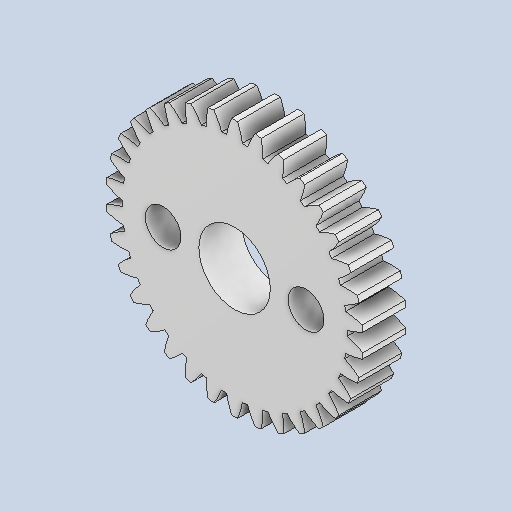
# Autodesk Inventor part: 平歯車1
Saved by Autodesk Inventor 2025.2 (Build 292293000, 293)
## iProperties
CustomPartVersion: 1
Created: 2025-01-10
Part Number: 平歯車1
Material: ABS プラスチック
Document SubType Name: Modeling
Designer: haruy
Categories: <?xml version="1.0" encoding="UTF-16"?> <MemberInstance><Categories><FamilyTemplate><FamilyTemplateParameter ValueType="xs:double" Id="1" ObjectReferenceKey="da_z" ObjectType="kUserParameterObject"/><FamilyTemplateParameter ValueType="xs:double" Id="2" ObjectReferenceKey="da_b" ObjectType="kUserParameterObject"/><FamilyTemplateParameter ValueType="xs:double" Id="3" ObjectReferenceKey="da_beta" ObjectType="kUserParameterObject"/><FamilyTemplateParameter ValueType="xs:double" Id="4" ObjectReferenceKey="da_da" ObjectType="kUserParameterObject"/><FamilyTemplateParameter ValueType="xs:double" Id="5" ObjectReferenceKey="da_aw" ObjectType="kUserParameterObject"/><FamilyTemplateParameter ValueType="xs:string" Id="6" ObjectReferenceKey="EAIAABAAAACIAQAAAAAAAIAAAAAAAAAA" ObjectType="83910656" SubObjectId="SurfaceGeometry"/></FamilyTemplate><ParamToTemplateMap><ParamToTemplate CategoryParameter="//CategoryParameter[@InternalName='046C89C9-8512-4d59-83FE-43B91F4F132A']" TemplateParameter="1"/><ParamToTemplate CategoryParameter="//CategoryParameter[@InternalName='2552DF32-E462-4b46-AEBF-C6C7768E72AC']" TemplateParameter="2"/><ParamToTemplate CategoryParameter="//CategoryParameter[@InternalName='C9EE641D-15FC-4fae-A226-E94C4372FDD7']" TemplateParameter="3"/><ParamToTemplate><ParamToTemplate CategoryParameter="//CategoryParameter[@InternalName='00B6519A-459B-49c7-AD84-2E56D39A5744']" ConstantValue="0.000000"/></ParamToTemplate><ParamToTemplate><ParamToTemplate CategoryParameter="//CategoryParameter[@InternalName='04B31F0E-C7A6-4894-AA32-9629BEFACF47']" ConstantValue="1.000000"/></ParamToTemplate><ParamToTemplate><ParamToTemplate CategoryParameter="//CategoryParameter[@InternalName='43CBEC2E-7847-49e7-A936-2F7889FCB2D9']" ConstantValue="0.250000"/></ParamToTemplate><ParamToTemplate><ParamToTemplate CategoryParameter="//CategoryParameter[@InternalName='B1EFC894-105D-4ebd-86BF-FA20ED196853']" ConstantValue="0.350000"/></ParamToTemplate><ParamToTemplate><ParamToTemplate CategoryParameter="//CategoryParameter[@InternalName='51175063-3D10-4879-93E8-6246FE8B403D']" ConstantValue="2060000000.000000"/></ParamToTemplate><ParamToTemplate><ParamToTemplate CategoryParameter="//CategoryParameter[@InternalName='A3A52E27-4454-46a9-B0BD-C932399B70AF']" ConstantValue="0.300000"/></ParamToTemplate><ParamToTemplate><ParamToTemplate CategoryParameter="//CategoryParameter[@InternalName='91B76062-C214-41d9-B1B9-14D2AB99603D']" ConstantValue="0.100000"/></ParamToTemplate><ParamToTemplate><ParamToTemplate CategoryParameter="//CategoryParameter[@InternalName='374E806E-8B8A-4dda-A9AA-1039D6500AD2']" ConstantValue="10.000000"/></ParamToTemplate><ParamToTemplate><ParamToTemplate CategoryParameter="//CategoryParameter[@InternalName='2D373A89-B862-43d6-8D0B-0CBF12AB9F6C']" ConstantValue="0.349066"/></ParamToTemplate><ParamToTemplate CategoryParameter="//CategoryParameter[@InternalName='37777632-D6A2-4fac-9D53-DB8ACD95C989']" TemplateParameter="4"/><ParamToTemplate CategoryParameter="//CategoryParameter[@InternalName='FD1017F1-B727-4f7e-9707-0F86F1FF9423']" TemplateParameter="5"/><ParamToTemplate><ParamToTemplate CategoryParameter="//CategoryParameter[@InternalName='9E1B4470-B2D3-4ff1-B813-535BB4CDF51A']" ConstantValue="3520000.000000"/></ParamToTemplate><ParamToTemplate><ParamToTemplate CategoryParameter="//CategoryParameter[@InternalName='F8452263-BFF6-458c-9FB1-07C4B99E95CD']" ConstantValue="11400000.000000"/></ParamToTemplate><ParamToTemplate><ParamToTemplate CategoryParameter="//CategoryParameter[@InternalName='3E3BB259-FD49-497f-8171-6EBC954A3479']" ConstantValue="2.000000"/></ParamToTemplate><ParamToTemplate CategoryParameter="//CategoryParameter[@InternalName='27C3BAF2-7550-4e4b-AE2C-0DB134B7D9B7']" TemplateParameter="6"/></ParamToTemplateMap><Category DisplayName="Gear" InternalName="DC85795E-93AB-48d5-8EEE-5A27447B64BD" Mnemonic="Gear"><CategoryParameter DisplayName="z" InternalName="046C89C9-8512-4d59-83FE-43B91F4F132A" Mnemonic="z"/><CategoryParameter DisplayName="b" InternalName="2552DF32-E462-4b46-AEBF-C6C7768E72AC" Mnemonic="b"/><CategoryParameter DisplayName="||b|" InternalName="C9EE641D-15FC-4fae-A226-E94C4372FDD7" Mnemonic="beta"/><CategoryParameter DisplayName="x" InternalName="00B6519A-459B-49c7-AD84-2E56D39A5744" Mnemonic="x"/><CategoryParameter DisplayName="a*" InternalName="04B31F0E-C7A6-4894-AA32-9629BEFACF47" Mnemonic="a"/><CategoryParameter DisplayName="c*" InternalName="43CBEC2E-7847-49e7-A936-2F7889FCB2D9" Mnemonic="c"/><CategoryParameter DisplayName="r|.f|*" InternalName="B1EFC894-105D-4ebd-86BF-FA20ED196853" Mnemonic="rf"/><CategoryParameter DisplayName="E" InternalName="51175063-3D10-4879-93E8-6246FE8B403D" Mnemonic="E"/><CategoryParameter DisplayName="||m|" InternalName="A3A52E27-4454-46a9-B0BD-C932399B70AF" Mnemonic="mi"/><Category DisplayName="SpurGear" InternalName="26C5A22E-A91E-4dfd-A3B3-23CCAFAE1764" Mnemonic="SpurGear"><CategoryParameter DisplayName="m" InternalName="91B76062-C214-41d9-B1B9-14D2AB99603D" Mnemonic="m"/><CategoryParameter DisplayName="P" InternalName="374E806E-8B8A-4dda-A9AA-1039D6500AD2" Mnemonic="PP"/><CategoryParameter DisplayName="||a|" InternalName="2D373A89-B862-43d6-8D0B-0CBF12AB9F6C" Mnemonic="alpha"/><CategoryParameter DisplayName="d|.a|" InternalName="37777632-D6A2-4fac-9D53-DB8ACD95C989" Mnemonic="da"/><CategoryParameter DisplayName="a|.w|" InternalName="FD1017F1-B727-4f7e-9707-0F86F1FF9423" Mnemonic="aw"/><CategoryParameter DisplayName="||s||.Flim|" InternalName="9E1B4470-B2D3-4ff1-B813-535BB4CDF51A" Mnemonic="sFlim"/><CategoryParameter DisplayName="||s||.Hlim|" InternalName="F8452263-BFF6-458c-9FB1-07C4B99E95CD" Mnemonic="sHlim"/><CategoryParameter DisplayName="タイプ" InternalName="3E3BB259-FD49-497f-8171-6EBC954A3479" Mnemonic="type"/><CategoryParameter DisplayName="PitchDiameter" InternalName="27C3BAF2-7550-4e4b-AE2C-0DB134B7D9B7" Mnemonic="IDS_PITCHDIAM"/></Category></Category></Categories></MemberInstance>
Density: 1.06 g/cm^3
Appearance: 滑らか - 白
Author: haruy
Autodesk Inventor part; units mm, degrees
sketch "Sketch1" plane through (0, 0, 0) normal (0, 0, 1) x (1, 0, 0)
  circle A0 centre (0, 0) radius 18
  dimension "d0" = 36
  constraints: 1 centre point
  measures "d0" diameter of A0
extrude "Extrusion1" add sketch "Sketch1" along normal blind 6
ref_plane "Work Plane2" through (0, 0, 3) normal (0, 0, 1) x (1, 0, 0)
sketch "Sketch2" plane through (0, 0, 0) normal (0, 0, -1) x (-1, 0, 0)
  circle A0 centre (0, 0) radius 18 projected
  circle A1 centre (0, 0) radius 17
  dimension "d3" = 34
  constraints: 1 centre point, 1 coincident
  measures "d3" diameter of A1
surface extrude "ピッチ円直径" sketch "Sketch2" against normal through all shown no curves A1
ref_plane "Work Plane8" through (0, 0, 0) normal (0.9957342, 0.0922684, 0) x (0, 0, 1)
ref_plane "Work Plane9" through (0, 0, 0) normal (1, 0, 0) x (0, 1, 0)
spur gear teeth "平歯車" teeth 34 pitch diameter 34 tip diameter 36 root diameter 31.5 face width 6 start plane through (0, 0, 0) normal (0, 0, -1) x (-1, 0, 0)
sketch "スケッチ3" plane through (0, 0, 6) normal (0, 0, 1) x (1, 0, 0)
  circle A0 centre (0, 0) radius 5
  circle A1 centre (0, 0) radius 10
  circle A2 centre (-10, 0) radius 2.5
  circle A3 centre (10, 0) radius 2.5
  dimension "d50" = 20
  dimension "d49" = 10
  dimension "d51" = 5
  dimension "d54" = 360
  constraints: 3 centre point, 2 coincident, 1 horizontal alignment, 7 other
  measures "d49" diameter of A0
  measures "d51" diameter of A2
extrude "押し出し2" cut sketch "スケッチ3" against normal blind 10 contours A0 | A1 A3 | A1 A3 | A2 A1 | A1 A2
sketch "スケッチ4" plane through (0, 0, 6) normal (0, 0, 1) x (1, 0, 0)
  circle A0 centre (10, 0) radius 2.5 projected
  circle A1 centre (-10, 0) radius 2.5 projected
  circle A2 centre (0, 0) radius 5 projected
  arc A3 (-3.7153, 17.6124) -> (-3.9591, 15.2443) centre (6.5578, 15.358) ccw projected
  arc A4 (-3.9591, 15.2443) -> (-4.6589, 15.0452) centre (0, 0) ccw projected
  arc A5 (-4.6589, 15.0452) -> (-6.1129, 16.9302) centre (-13.6605, 9.6054) ccw projected
  arc A6 (-6.1129, 16.9302) -> (-6.8883, 16.6298) centre (0, 0) ccw projected
  arc A7 (-6.8883, 16.6298) -> (-6.6929, 14.2572) centre (3.6241, 16.3015) ccw projected
  arc A8 (-6.6929, 14.2572) -> (-7.3442, 13.9329) centre (0, 0) ccw projected
  arc A9 (-7.3442, 13.9329) -> (-9.1198, 15.5187) centre (-15.1929, 6.9317) ccw projected
  arc A10 (-9.1198, 15.5187) -> (-9.8267, 15.081) centre (0, 0) ccw projected
  arc A11 (-9.8267, 15.081) -> (-9.1987, 12.7847) centre (0.567, 16.6898) ccw projected
  arc A12 (-9.1987, 12.7847) -> (-9.7793, 12.3462) centre (0, 0) ccw projected
  arc A13 (-9.7793, 12.3462) -> (-11.816, 13.5787) centre (-16.2079, 4.022) ccw projected
  arc A14 (-11.816, 13.5787) -> (-12.4305, 13.0185) centre (0, 0) ccw projected
  arc A15 (-12.4305, 13.0185) -> (-11.3912, 10.8767) centre (-2.5094, 16.5098) ccw projected
  arc A16 (-11.3912, 10.8767) -> (-11.8814, 10.339) centre (0, 0) ccw projected
  arc A17 (-11.8814, 10.339) -> (-14.1099, 11.1763) centre (-16.6709, 0.9753) ccw projected
  arc A18 (-14.1099, 11.1763) -> (-14.611, 10.5127) centre (0, 0) ccw projected
  arc A19 (-14.611, 10.5127) -> (-13.1958, 8.5984) centre (-5.5003, 15.7676) ccw projected
  arc A20 (-13.1958, 8.5984) -> (-13.5789, 7.9798) centre (0, 0) ccw projected
  arc A21 (-13.5789, 7.9798) -> (-15.9233, 8.3933) centre (-16.5663, -2.1046) ccw projected
  arc A22 (-15.9233, 8.3933) -> (-16.294, 7.649) centre (0, 0) ccw projected
  arc A23 (-16.294, 7.649) -> (-14.5511, 6.0273) centre (-8.304, 14.4885) ccw projected
  arc A24 (-14.5511, 6.0273) -> (-14.8139, 5.3488) centre (0, 0) ccw projected
  arc A25 (-14.8139, 5.3488) -> (-17.1945, 5.3245) centre (-15.8975, -5.1128) ccw projected
  arc A26 (-17.1945, 5.3245) -> (-17.422, 4.5247) centre (0, 0) ccw projected
  arc A27 (-17.422, 4.5247) -> (-15.4108, 3.2509) centre (-10.8248, 12.7159) ccw projected
  arc A28 (-15.4108, 3.2509) -> (-15.5445, 2.5357) centre (0, 0) ccw projected
  arc A29 (-15.5445, 2.5357) -> (-17.8801, 2.0744) centre (-14.6874, -7.9469) ccw projected
  arc A30 (-17.8801, 2.0744) -> (-17.9568, 1.2464) centre (0, 0) ccw projected
  arc A31 (-17.9568, 1.2464) -> (-15.7458, 0.3638) centre (-12.9771, 10.5104) ccw projected
  arc A32 (-15.7458, 0.3638) -> (-15.7458, -0.3638) centre (0, 0) ccw projected
  arc A33 (-15.7458, -0.3638) -> (-17.9568, -1.2464) centre (-12.9771, -10.5104) ccw projected
  arc A34 (-17.9568, -1.2464) -> (-17.8801, -2.0744) centre (0, 0) ccw projected
  arc A35 (-17.8801, -2.0744) -> (-15.5445, -2.5357) centre (-14.6874, 7.9469) ccw projected
  arc A36 (-15.5445, -2.5357) -> (-15.4108, -3.2509) centre (0, 0) ccw projected
  arc A37 (-15.4108, -3.2509) -> (-17.422, -4.5247) centre (-10.8248, -12.7159) ccw projected
  arc A38 (-17.422, -4.5247) -> (-17.1945, -5.3245) centre (0, 0) ccw projected
  arc A39 (-17.1945, -5.3245) -> (-14.8139, -5.3488) centre (-15.8975, 5.1128) ccw projected
  arc A40 (-14.8139, -5.3488) -> (-14.5511, -6.0273) centre (0, 0) ccw projected
  arc A41 (-14.5511, -6.0273) -> (-16.294, -7.649) centre (-8.304, -14.4885) ccw projected
  arc A42 (-16.294, -7.649) -> (-15.9233, -8.3933) centre (0, 0) ccw projected
  arc A43 (-15.9233, -8.3933) -> (-13.5789, -7.9798) centre (-16.5663, 2.1046) ccw projected
  arc A44 (-13.5789, -7.9798) -> (-13.1958, -8.5984) centre (0, 0) ccw projected
  arc A45 (-13.1958, -8.5984) -> (-14.611, -10.5127) centre (-5.5003, -15.7676) ccw projected
  arc A46 (-14.611, -10.5127) -> (-14.1099, -11.1763) centre (0, 0) ccw projected
  arc A47 (-14.1099, -11.1763) -> (-11.8814, -10.339) centre (-16.6709, -0.9753) ccw projected
  arc A48 (-11.8814, -10.339) -> (-11.3912, -10.8767) centre (0, 0) ccw projected
  arc A49 (-11.3912, -10.8767) -> (-12.4305, -13.0185) centre (-2.5094, -16.5098) ccw projected
  arc A50 (-12.4305, -13.0185) -> (-11.816, -13.5787) centre (0, 0) ccw projected
  arc A51 (-11.816, -13.5787) -> (-9.7793, -12.3462) centre (-16.2079, -4.022) ccw projected
  arc A52 (-9.7793, -12.3462) -> (-9.1987, -12.7847) centre (0, 0) ccw projected
  arc A53 (-9.1987, -12.7847) -> (-9.8267, -15.081) centre (0.567, -16.6898) ccw projected
  arc A54 (-9.8267, -15.081) -> (-9.1198, -15.5187) centre (0, 0) ccw projected
  arc A55 (-9.1198, -15.5187) -> (-7.3442, -13.9329) centre (-15.1929, -6.9317) ccw projected
  arc A56 (-7.3442, -13.9329) -> (-6.6929, -14.2572) centre (0, 0) ccw projected
  arc A57 (-6.6929, -14.2572) -> (-6.8883, -16.6298) centre (3.6241, -16.3015) ccw projected
  arc A58 (-6.8883, -16.6298) -> (-6.1129, -16.9302) centre (0, 0) ccw projected
  arc A59 (-6.1129, -16.9302) -> (-4.6589, -15.0452) centre (-13.6605, -9.6054) ccw projected
  arc A60 (-4.6589, -15.0452) -> (-3.9591, -15.2443) centre (0, 0) ccw projected
  arc A61 (-3.9591, -15.2443) -> (-3.7153, -17.6124) centre (6.5578, -15.358) ccw projected
  arc A62 (-3.7153, -17.6124) -> (-2.8979, -17.7652) centre (0, 0) ccw projected
  arc A63 (-2.8979, -17.7652) -> (-1.8151, -15.6451) centre (-11.6629, -11.9519) ccw projected
  arc A64 (-1.8151, -15.6451) -> (-1.0906, -15.7122) centre (0, 0) ccw projected
  arc A65 (-1.0906, -15.7122) -> (-0.4158, -17.9952) centre (9.2682, -13.8915) ccw projected
  arc A66 (-0.4158, -17.9952) -> (0.4158, -17.9952) centre (0, 0) ccw projected
  arc A67 (0.4158, -17.9952) -> (1.0906, -15.7122) centre (-9.2682, -13.8915) ccw projected
  arc A68 (1.0906, -15.7122) -> (1.8151, -15.6451) centre (0, 0) ccw projected
  arc A69 (1.8151, -15.6451) -> (2.8979, -17.7652) centre (11.6629, -11.9519) ccw projected
  arc A70 (2.8979, -17.7652) -> (3.7153, -17.6124) centre (0, 0) ccw projected
  arc A71 (3.7153, -17.6124) -> (3.9591, -15.2443) centre (-6.5578, -15.358) ccw projected
  arc A72 (3.9591, -15.2443) -> (4.6589, -15.0452) centre (0, 0) ccw projected
  arc A73 (4.6589, -15.0452) -> (6.1129, -16.9302) centre (13.6605, -9.6054) ccw projected
  arc A74 (6.1129, -16.9302) -> (6.8883, -16.6298) centre (0, 0) ccw projected
  arc A75 (6.8883, -16.6298) -> (6.6929, -14.2572) centre (-3.6241, -16.3015) ccw projected
  arc A76 (6.6929, -14.2572) -> (7.3442, -13.9329) centre (0, 0) ccw projected
  arc A77 (7.3442, -13.9329) -> (9.1198, -15.5187) centre (15.1929, -6.9317) ccw projected
  arc A78 (9.1198, -15.5187) -> (9.8267, -15.081) centre (0, 0) ccw projected
  arc A79 (9.8267, -15.081) -> (9.1987, -12.7847) centre (-0.567, -16.6898) ccw projected
  arc A80 (9.1987, -12.7847) -> (9.7793, -12.3462) centre (0, 0) ccw projected
  arc A81 (9.7793, -12.3462) -> (11.816, -13.5787) centre (16.2079, -4.022) ccw projected
  arc A82 (11.816, -13.5787) -> (12.4305, -13.0185) centre (0, 0) ccw projected
  arc A83 (12.4305, -13.0185) -> (11.3912, -10.8767) centre (2.5094, -16.5098) ccw projected
  arc A84 (11.3912, -10.8767) -> (11.8814, -10.339) centre (0, 0) ccw projected
  arc A85 (11.8814, -10.339) -> (14.1099, -11.1763) centre (16.6709, -0.9753) ccw projected
  arc A86 (14.1099, -11.1763) -> (14.611, -10.5127) centre (0, 0) ccw projected
  arc A87 (14.611, -10.5127) -> (13.1958, -8.5984) centre (5.5003, -15.7676) ccw projected
  arc A88 (13.1958, -8.5984) -> (13.5789, -7.9798) centre (0, 0) ccw projected
  arc A89 (13.5789, -7.9798) -> (15.9233, -8.3933) centre (16.5663, 2.1046) ccw projected
  arc A90 (15.9233, -8.3933) -> (16.294, -7.649) centre (0, 0) ccw projected
  arc A91 (16.294, -7.649) -> (14.5511, -6.0273) centre (8.304, -14.4885) ccw projected
  arc A92 (14.5511, -6.0273) -> (14.8139, -5.3488) centre (0, 0) ccw projected
  arc A93 (14.8139, -5.3488) -> (17.1945, -5.3245) centre (15.8975, 5.1128) ccw projected
  arc A94 (17.1945, -5.3245) -> (17.422, -4.5247) centre (0, 0) ccw projected
  arc A95 (17.422, -4.5247) -> (15.4108, -3.2509) centre (10.8248, -12.7159) ccw projected
  arc A96 (15.4108, -3.2509) -> (15.5445, -2.5357) centre (0, 0) ccw projected
  arc A97 (15.5445, -2.5357) -> (17.8801, -2.0744) centre (14.6874, 7.9469) ccw projected
  arc A98 (17.8801, -2.0744) -> (17.9568, -1.2464) centre (0, 0) ccw projected
  arc A99 (17.9568, -1.2464) -> (15.7458, -0.3638) centre (12.9771, -10.5104) ccw projected
  arc A100 (15.7458, -0.3638) -> (15.7458, 0.3638) centre (0, 0) ccw projected
  arc A101 (15.7458, 0.3638) -> (17.9568, 1.2464) centre (12.9771, 10.5104) ccw projected
  arc A102 (17.9568, 1.2464) -> (17.8801, 2.0744) centre (0, 0) ccw projected
  arc A103 (17.8801, 2.0744) -> (15.5445, 2.5357) centre (14.6874, -7.9469) ccw projected
  arc A104 (15.5445, 2.5357) -> (15.4108, 3.2509) centre (0, 0) ccw projected
  arc A105 (15.4108, 3.2509) -> (17.422, 4.5247) centre (10.8248, 12.7159) ccw projected
  arc A106 (17.422, 4.5247) -> (17.1945, 5.3245) centre (0, 0) ccw projected
  arc A107 (17.1945, 5.3245) -> (14.8139, 5.3488) centre (15.8975, -5.1128) ccw projected
  arc A108 (14.8139, 5.3488) -> (14.5511, 6.0273) centre (0, 0) ccw projected
  arc A109 (14.5511, 6.0273) -> (16.294, 7.649) centre (8.304, 14.4885) ccw projected
  arc A110 (16.294, 7.649) -> (15.9233, 8.3933) centre (0, 0) ccw projected
  arc A111 (15.9233, 8.3933) -> (13.5789, 7.9798) centre (16.5663, -2.1046) ccw projected
  arc A112 (13.5789, 7.9798) -> (13.1958, 8.5984) centre (0, 0) ccw projected
  arc A113 (13.1958, 8.5984) -> (14.611, 10.5127) centre (5.5003, 15.7676) ccw projected
  arc A114 (14.611, 10.5127) -> (14.1099, 11.1763) centre (0, 0) ccw projected
  arc A115 (14.1099, 11.1763) -> (11.8814, 10.339) centre (16.6709, 0.9753) ccw projected
  arc A116 (11.8814, 10.339) -> (11.3912, 10.8767) centre (0, 0) ccw projected
  arc A117 (11.3912, 10.8767) -> (12.4305, 13.0185) centre (2.5094, 16.5098) ccw projected
  arc A118 (12.4305, 13.0185) -> (11.816, 13.5787) centre (0, 0) ccw projected
  arc A119 (11.816, 13.5787) -> (9.7793, 12.3462) centre (16.2079, 4.022) ccw projected
  arc A120 (9.7793, 12.3462) -> (9.1987, 12.7847) centre (0, 0) ccw projected
  arc A121 (9.1987, 12.7847) -> (9.8267, 15.081) centre (-0.567, 16.6898) ccw projected
  arc A122 (9.8267, 15.081) -> (9.1198, 15.5187) centre (0, 0) ccw projected
  arc A123 (9.1198, 15.5187) -> (7.3442, 13.9329) centre (15.1929, 6.9317) ccw projected
  arc A124 (7.3442, 13.9329) -> (6.6929, 14.2572) centre (0, 0) ccw projected
  arc A125 (6.6929, 14.2572) -> (6.8883, 16.6298) centre (-3.6241, 16.3015) ccw projected
  arc A126 (6.8883, 16.6298) -> (6.1129, 16.9302) centre (0, 0) ccw projected
  arc A127 (6.1129, 16.9302) -> (4.6589, 15.0452) centre (13.6605, 9.6054) ccw projected
  arc A128 (4.6589, 15.0452) -> (3.9591, 15.2443) centre (0, 0) ccw projected
  arc A129 (3.9591, 15.2443) -> (3.7153, 17.6124) centre (-6.5578, 15.358) ccw projected
  arc A130 (3.7153, 17.6124) -> (2.8979, 17.7652) centre (0, 0) ccw projected
  arc A131 (2.8979, 17.7652) -> (1.8151, 15.6451) centre (11.6629, 11.9519) ccw projected
  arc A132 (1.8151, 15.6451) -> (1.0906, 15.7122) centre (0, 0) ccw projected
  arc A133 (1.0906, 15.7122) -> (0.4158, 17.9952) centre (-9.2682, 13.8915) ccw projected
  arc A134 (0.4158, 17.9952) -> (-0.4158, 17.9952) centre (0, 0) ccw projected
  arc A135 (-0.4158, 17.9952) -> (-1.0906, 15.7122) centre (9.2682, 13.8915) ccw projected
  arc A136 (-1.0906, 15.7122) -> (-1.8151, 15.6451) centre (0, 0) ccw projected
  arc A137 (-1.8151, 15.6451) -> (-2.8979, 17.7652) centre (-11.6629, 11.9519) ccw projected
  arc A138 (-2.8979, 17.7652) -> (-3.7153, 17.6124) centre (0, 0) ccw projected
equation "\"d0\" = da_da"
equation "\"d1\" = da_b"
equation "\"d3\" = da_d"
equation "\"d16\" = da_aw"
equation "\"d43\" = da_aw"
equation "\"d46\" = da_aw"
equation "\"da_da\" = 36"
equation "\"da_b\" = 6"
equation "\"da_d\" = 34"
equation "\"da_aw\" = 33"
body "Solid1"
body "Srf1"
